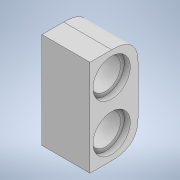
# Autodesk Inventor part: apoio_array
Saved by Autodesk Inventor 2020 (Build 240168000, 168)
## iProperties
Created: 2020-04-22
Part Number: apoio_array
Material: Genérico
Document SubType Name: Modeling
Designer: gi-se
Density: 1 g/cm^3
Appearance: Padrão
Author: gi-se
## iProperties of the stored document _3DPrint.ipt
Created: 2020-06-03
Part Number: _3DPrint
Material: Genérico
Document SubType Name: Modeling
Designer: gi-se
Density: 1 g/cm^3
Appearance: Padrão
Author: gi-se
Autodesk Inventor part; units mm, degrees
ref_plane "YZ Plane" through (0, 0, 0) normal (1, 0, 0) x (0, 1, 0)
ref_plane "XZ Plane" through (0, 0, 0) normal (0, 1, 0) x (-1, 0, 0)
ref_plane "XY Plane" through (0, 0, 0) normal (0, 0, 1) x (1, 0, 0)
sketch "Esboço1" plane through (0, 0, 0) normal (0, 0, 1) x (1, 0, 0)
  line L0 (16, -12) -> (8, -12)
  line L1 (8, -12) -> (8, 4)
  line L2 (8, 4) -> (16, 4)
  line L3 (16, 4) -> (16, -12)
  point P0 (0, 0)
  dimension "d0" = 8
  dimension "d1" = 16
  constraints: 8 end point, 2 parallel, 1 horizontal, 1 perpendicular
  measures "d0" distance of L1.end L2.end
  measures "d1" distance of L0.end L1.end
extrude "Extrusão1" add sketch "Esboço1" against normal blind 8
sketch "Esboço3" plane through (8, -12, 0) normal (-1, 0, 0) x (0, 0, 1)
  circle A0 centre (-3.6, 4) radius 2.4 projected
  circle A1 centre (-3.6, 12) radius 2.4 projected
  line L0 (0, 0) -> (-8, 0) projected
  line L1 (-3.6, 0) -> (-8, 0) construction
  line L2 (-8, 16) -> (-8, 0) projected
  line L3 (-8, 0) -> (-8, 4) construction
  spline S0 degree 2 poles (-3.6, 0) (-8, 0) (-8, 4) knots 1 1 1 2 2 2
  line L4 (0, 16) -> (-8, 16) projected
  line L5 (-3.6, 16) -> (-8, 16) construction
  line L6 (-8, 16) -> (-8, 12) construction
  spline S1 degree 2 poles (-3.6, 16) (-8, 16) (-8, 12) knots 1 1 1 2 2 2
  circle A2 centre (-3.6, 12) radius 2.5
  circle A3 centre (-3.6, 4) radius 2.5
  point P0 (0, 12)
  dimension "d14" = 5
  dimension "d15" = 5
  constraints: 4 coincident, 4 point on line, 2 centre point, 2 collinear, 6 other
  measures "d14" diameter of A2
  measures "d15" diameter of A3
extrude "Extrusão3" cut sketch "Esboço3" against normal blind 8 contours A0 | A1 | L2 L4 S1 | L0 L2 S0 | A2 | A3
sketch "Esboço4" plane through (8, -12, 0) normal (-1, 0, 0) x (0, 0, 1)
  circle A0 centre (-3.6, 12) radius 3.1 projected
  circle A1 centre (-3.6, 4) radius 3.1 projected
  point P0 (0, 12)
extrude "Extrusão4" cut sketch "Esboço4" against normal blind 1
sketch "Esboço5" plane through (16, -12, 0) normal (1, 0, 0) x (0, 0, -1)
  circle A0 centre (3.6, 12) radius 3.1 projected
  circle A1 centre (3.6, 4) radius 3.1 projected
  point P0 (0, 12)
extrude "Extrusão5" cut sketch "Esboço5" against normal blind 1
